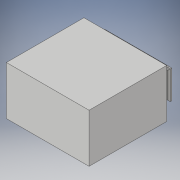
# Autodesk Inventor part: Power Socket Insert v1
Saved by Autodesk Inventor 2019 (Build 230136000, 136)
## iProperties
Created: 2021-08-06
Part Number: Power Socket Insert v1
Material: Generic
Document SubType Name: Modeling
Designer: Lix
Density: 1 g/cm^3
Appearance: Default
Author: Lix
Autodesk Inventor part; units mm, degrees
ref_plane "YZ Plane" through (0, 0, 0) normal (1, 0, 0) x (0, 1, 0)
ref_plane "XZ Plane" through (0, 0, 0) normal (0, 1, 0) x (-1, 0, 0)
ref_plane "XY Plane" through (0, 0, 0) normal (0, 0, 1) x (1, 0, 0)
sketch "Sketch1" plane through (0, 0, 0) normal (0, 0, 1) x (1, 0, 0)
  line L0 (-21.65, 9.15) -> (21.65, 9.15)
  line L1 (21.65, 9.15) -> (21.65, -9.15)
  line L2 (21.65, -9.15) -> (-21.65, -9.15)
  line L3 (-21.65, -9.15) -> (-21.65, 9.15)
  line L4 (-21.65, 9.15) -> (21.65, -9.15) construction
  line L5 (21.65, 9.15) -> (-21.65, -9.15) construction
  point P0 (0, 0)
  dimension "d0" = 43.3
  dimension "d1" = 18.3
  constraints: 12 end point, 2 midpoint, 2 parallel, 1 horizontal, 1 perpendicular
  measures "d0" distance of L0.start L0.end
  measures "d1" distance of L0.end L1.end
extrude "Extrusion1" add sketch "Sketch1" along normal blind 2
sketch "Sketch2" plane through (0, 0, 2) normal (0, 0, 1) x (1, 0, 0)
  line L0 (-19.15, 5.9) -> (19.15, 5.9)
  line L1 (19.15, 5.9) -> (19.15, -5.9)
  line L2 (19.15, -5.9) -> (-19.15, -5.9)
  line L3 (-19.15, -5.9) -> (-19.15, 5.9)
  line L4 (-19.15, 5.9) -> (19.15, -5.9) construction
  line L5 (19.15, 5.9) -> (-19.15, -5.9) construction
  point P0 (0, 0)
  dimension "d4" = 38.3
  dimension "d5" = 11.8
  constraints: 12 end point, 2 midpoint, 2 parallel, 1 horizontal, 1 perpendicular
  measures "d4" distance of L1.end L2.end
  measures "d5" distance of L0.end L1.end
extrude "Extrusion2" add sketch "Sketch2" along normal blind 2.5
chamfer "Chamfer1" distance 1 angle 45 4 edges at (0, -9.15, 2) (21.65, 0, 2) (-21.65, 0, 2) (0, 9.15, 2)
sketch "Sketch3" plane through (0, 0, 4.5) normal (0, 0, 1) x (1, 0, 0)
  line L0 (22.8185, -17.9) -> (-30.4815, -17.9)
  line L1 (-30.4815, -17.9) -> (-30.4815, 13.4)
  line L2 (-30.4815, 13.4) -> (22.8185, 13.4)
  line L3 (22.8185, 13.4) -> (22.8185, -17.9)
  line L4 (-30.4815, -17.9) -> (22.8185, 13.4) construction
  line L5 (19.15, 5.9) -> (-19.15, 5.9) projected
  line L6 (-19.15, -5.9) -> (19.15, -5.9) projected
  point P0 (0, 0)
  dimension "d11" = 53.3
  dimension "d12" = 7.5
  dimension "d13" = 12
  constraints: 10 end point, 2 parallel, 1 horizontal, 1 perpendicular, 1 point on line
  measures "d11" distance of L0.start L0.end
  measures "d12" distance between parallel lines of L2 L5
  measures "d13" distance between parallel lines of L0 L6
extrude "Extrusion3" add sketch "Sketch3" along normal blind 50
body "Solid1"
